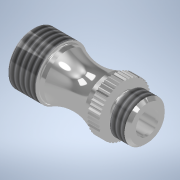
# Autodesk Inventor part: YTP-AP-E02-R1.0
Saved by Autodesk Inventor 2020.4 (Build 244396000, 396)
## iProperties
RuleStatus: InUse
AfterDocNew0: iPropertyEnforcement
BeforeDocSave0: Materialprüfung
Created: 2021-08-29
Part Number: YTP-AP-E02-R1.0
Project: Airbrush
Material: Messing, weicher Gelbton, geschweißt
Description: Luftventilgehaeuse
Document SubType Name: Modeling
Designer: Uwe Wieser
Mass: 4.97016 g
Surface Area: 9.3287 cm^2
Volume: 0.584724 cm^3
Density: 8.5 g/cm^3
Appearance: Chrom - poliert
Werkstoff: 1.4301
Author: Uwe Wieser
Autodesk Inventor part; units mm, degrees
ref_plane "YZ Plane" through (0, 0, 0) normal (1, 0, 0) x (0, 1, 0)
ref_plane "XZ Plane" through (0, 0, 0) normal (0, 1, 0) x (-1, 0, 0)
ref_plane "XY Plane" through (0, 0, 0) normal (0, 0, 1) x (1, 0, 0)
sketch "Skizze1" plane through (0, 0, 0) normal (0, 0, 1) x (1, 0, 0)
  line L0 (-15, 4.5) -> (-20, 4.5)
  line L1 (-14, 4) -> (-15, 4)
  arc A0 (-14, 4) -> (-7, 4) centre (-10.5, 12.2916) ccw
  line L2 (-6, 4) -> (-7, 4)
  line L3 (-4, 4.5) -> (-6, 4.5)
  line L4 (-4, 4.5) -> (-4, 2.7)
  line L5 (-3, 2.7) -> (-4, 2.7)
  line L6 (-0.5, 3.5) -> (-3, 3.5)
  line L7 (0, 3) -> (-0.5, 3.5)
  line L8 (-0.5, 2) -> (0, 2)
  line L9 (-0.5, 2.25) -> (-16, 2.25)
  line L10 (-16, 3) -> (-16, 2.25)
  line L11 (-16, 3) -> (-20, 3)
  line L12 (0, -2.4583) -> (0, 14.7499) projected
  line L13 (-24, 0) -> (4, 0) projected
  line L14 (-0.5, 2.25) -> (-0.5, 2)
  line L15 (-3, 3.5) -> (-3, 2.7)
  line L16 (-6, 4.5) -> (-6, 4)
  line L17 (0, 3) -> (0, 2)
  line L18 (-15, 4.5) -> (-15, 4)
  line L19 (-20, 4.5) -> (-20, 3)
  point P0 (0, 0)
  dimension "d0" = 20
  dimension "d1" = 4
  dimension "d2" = 1
  dimension "d3" = 0.5
  dimension "d4" = 2
  dimension "d5" = 1
  dimension "d6" = 2.5
  dimension "d7" = 0.5
  dimension "d8" = 1
  dimension "d9" = 5
  dimension "d10" = 1
  dimension "d11" = 9
  dimension "d12" = 15.5
  dimension "d13" = 6
  dimension "d14" = 4.5
  dimension "d15" = 4
  dimension "d16" = 7
  dimension "d17" = 5.4
  dimension "d18" = 9
  dimension "d19" = 8
  dimension "d20" = 8
  dimension "d21" = 9
  dimension "d22" = 10.5
  constraints: 36 end point, 3 parallel, 2 point on circle, 2 point on line, 1 centre point, 1 collinear
  measures "d0" distance between parallel lines of L12 L19
  measures "d1" distance of L11.start L11.end
  measures "d2" distance of L7.start L8.end
  measures "d3" distance of L8.start L8.end
  measures "d4" distance of L3.start L3.end
  measures "d5" distance of L5.start L4.end
  measures "d6" distance of L6.start L6.end
  measures "d7" horizontal distance of L7.start L7.end
  measures "d8" distance of L2.start L2.end
  measures "d9" distance of L0.start L0.end
  measures "d10" distance of L1.start L1.end
  measures "d11" radius of A0
  measures "d12" distance of L9.start L9.end
  measures "d13" diameter of L11 L13
  measures "d14" diameter of L9 L13
  measures "d15" diameter of L8 L13
  measures "d16" diameter of L6 L13
  measures "d17" diameter of L5 L13
  measures "d18" diameter of L3 L13
  measures "d19" diameter of L2 L13
  measures "d20" diameter of L1 L13
  measures "d21" diameter of L0 L13
  measures "d22" distance from line of L12 A0.centre
revolve "Umdrehung1" add sketch "Skizze1" angle 360 about axis through (-10, 0, 0) along (1, 0, 0)
thread "Gewinde1" size "G7.723x0.907" designation "G 1/16" class "A" standard "ISO Pipe Threads" full length
sketch "Skizze2" plane through (-6, 0, 0) normal (-1, 0, 0) x (0, 0, 1)
  circle A0 centre (0, 0) radius 3.5 projected
  circle A1 centre (0, 0) radius 4.5 projected
  line L0 (0, -6.3) -> (0, 6.3) projected
  line L1 (0, 4.3) -> (0.25, 4.4931)
  line L2 (0, 4.3) -> (-0.25, 4.4931)
  dimension "d26" = 4.3
  dimension "d27" = 0.5
  constraints: 4 end point, 2 point on circle, 1 point on line, 1 symmetric about line
  measures "d26" distance of point (0, 0) L1.start
  measures "d27" distance of L2.end L1.end
extrude "Extrusion1" cut sketch "Skizze2" against normal up to surface (2 mm away) contours L2 A1 L0 | L0 A1 L1
pattern_circular "Runde Anordnung1" count 45 over 360 about axis through (-10, 0, 0) along (1, 0, 0) of "Extrusion1"
chamfer "Fase1" distance 0.3 angle 45 2 edges at (-20, -3, 0) (-20, -4.5, 0)
fillet "Rundung1" radius 0.3 4 edges at (-4, -2.7, 0) (-3, -2.7, 0) (-6, -4, 0) (-15, -4, 0)
thread "Gewinde3" size "G9.728x0.907" designation "G 1/8" class "A" standard "ISO Pipe Threads" full length
